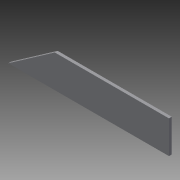
# Autodesk Inventor part: Left Forearm
Saved by Autodesk Inventor 2014 (Build 180170000, 170)
## iProperties
Created: 2015-08-01
Part Number: Left Forearm
Material: Generic
Document SubType Name: Modeling
Designer: Devon
Density: 1 g/cm^3
Appearance: Default
Author: Devon
Autodesk Inventor part; units mm, degrees
ref_plane "YZ Plane" through (0, 0, 0) normal (1, 0, 0) x (0, 1, 0)
ref_plane "XZ Plane" through (0, 0, 0) normal (0, 1, 0) x (-1, 0, 0)
ref_plane "XY Plane" through (0, 0, 0) normal (0, 0, 1) x (1, 0, 0)
sketch "Sketch1" plane through (0, 0, 0) normal (0, 0, 1) x (1, 0, 0)
  line L0 (-26.4763, -7.5222) -> (152.9112, -7.5222)
  line L1 (-26.4763, -7.5222) -> (25.5399, 28.8999)
  line L2 (-26.4763, -7.5222) -> (37.0237, -7.5222) construction
  line L3 (25.5399, 28.8999) -> (152.9112, 28.8999)
  line L4 (152.9112, 28.8999) -> (152.9112, -7.5222)
  point P0 (0, 0)
  dimension "d0" = 179.3875
  dimension "d2" = 63.5
  dimension "d3" = 35
  constraints: 10 end point, 2 horizontal, 1 equal length, 1 perpendicular
  measures "d0" distance of L0.start L0.end
  measures "d2" distance of L0.start L1.end
  measures "d3" angle of L2 L1
extrude "Extrusion1" add sketch "Sketch1" along normal blind 3.175
body "Solid1"
